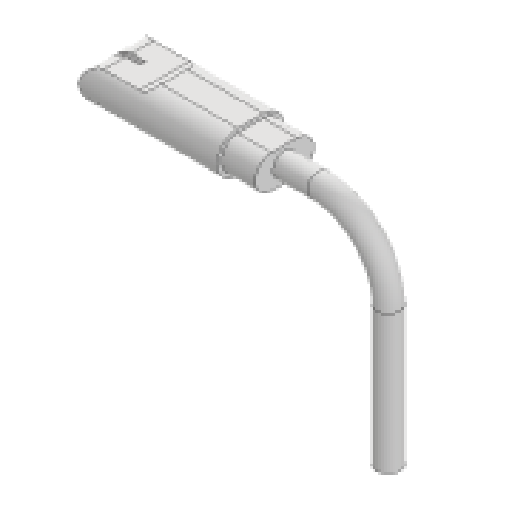
# Autodesk Inventor part: 基座
Saved by Autodesk Inventor 2025.2 (Build 292293000, 293)
## iProperties
Created: 2025-07-22
Part Number: 基座
Material: 一般
Document SubType Name: Modeling
Designer: jna1j
Density: 1 g/cm^3
Appearance: 預設
Author: jna1j
Autodesk Inventor part; units mm, degrees
ref_plane "YZ Plane" through (0, 0, 0) normal (1, 0, 0) x (0, 1, 0)
ref_plane "XZ Plane" through (0, 0, 0) normal (0, 1, 0) x (-1, 0, 0)
ref_plane "XY Plane" through (0, 0, 0) normal (0, 0, 1) x (1, 0, 0)
sketch "草圖1" plane through (0, 0, 0) normal (1, 0, 0) x (0, 1, 0)
  line L0 (-2.97, -1.859) -> (2.97, -1.859)
  line L1 (2.97, -1.859) -> (2.97, 1.859)
  line L2 (2.97, 1.859) -> (-2.97, 1.859)
  line L3 (-2.97, 1.859) -> (-2.97, -1.859)
  line L4 (-2.97, -1.859) -> (2.97, 1.859) construction
  line L5 (2.97, -1.859) -> (-2.97, 1.859) construction
  circle A0 centre (0, 1.859) radius 2.97
  circle A1 centre (0, -1.859) radius 2.97
  line L6 (-2.2651, -3.78) -> (-2.2651, 3.78) construction
  point P0 (0, 0)
  point P1 (-2.97, 1.859)
  dimension "d0" = 7.56
  dimension "d1" = 5.94
  constraints: 14 end point, 4 midpoint, 4 point on circle, 2 centre point, 2 parallel, 1 horizontal, 1 perpendicular, 1 vertical
  measures "d0" distance of L6.start L6.end
  measures "d1" distance of L1.end L2.end
extrude "擠出1" add sketch "草圖1" along normal blind 20
sketch "草圖2" plane through (0, 0, 0) normal (0, 0, 1) x (1, 0, 0)
  line L0 (0, 2.4) -> (9, 2.4)
  line L1 (9, 2.4) -> (9, -2.4)
  line L2 (9, -2.4) -> (0, -2.4)
  line L3 (0, -2.4) -> (0, 2.4)
  line L4 (0, -2.97) -> (0, 2.97) projected
  circle A0 centre (2.4, 0) radius 2.4
  line L5 (9, 5) -> (20, 5)
  line L6 (20, 5) -> (20, -5)
  line L7 (20, -5) -> (9, -5)
  line L8 (9, -5) -> (9, 5)
  line L9 (0, -2.97) -> (0, 2.97) projected
  line L10 (0, 2.97) -> (20, 2.97) projected
  line L11 (20, -2.97) -> (20, 2.97) projected
  line L12 (0, -2.97) -> (20, -2.97) projected
  arc A1 (7.6018, 2.4) -> (9, 2.97) centre (7.6018, 4.4) ccw
  arc A2 (9, -2.97) -> (7.6018, -2.4) centre (7.6018, -4.4) ccw
  point P0 (0, 0)
  point P1 (0, 0)
  point P2 (9, 0)
  point P3 (2.4, 2.4)
  point P4 (2.4, -2.4)
  dimension "d4" = 4.8
  dimension "d5" = 9
  dimension "d6" = 2
  dimension "d7" = 2
  constraints: 16 end point, 6 point on line, 5 tangent, 4 midpoint, 4 parallel, 4 point on circle, 3 centre point, 2 horizontal, 2 perpendicular
  measures "d4" distance of L2.end L0.start
  measures "d5" distance of L1.end L2.end
  measures "d6" radius of A2
  measures "d7" radius of A1
extrude "擠出2" cut sketch "草圖2" along normal mid plane 20 contours A1 L8 L0 | L0 L1 L2 A0 | L8 L10 L6 L12 L1 | A0 | L8 L5 L6 L10 | L8 A2 L2 | L12 L6 L7 L8 keep common part
sketch "草圖3" plane through (0, 0, 0) normal (0, 0, 1) x (1, 0, 0)
  line L0 (-0.1991, -1.7797) -> (-0.0573, 1.9709) projected
  arc A0 (-0.1991, -1.7797) -> (-0.0573, 1.9709) centre (2.4, 0) ccw projected
  point P0 (0, 0)
extrude "擠出3" cut sketch "草圖3" along normal mid plane 0.84
sketch "草圖4" plane through (20, 0, 0) normal (1, 0, 0) x (0, 0, -1)
  line L0 (1.859, 2.97) -> (-1.859, 2.97) projected
  arc A0 (-1.859, 2.97) -> (-1.859, -2.97) centre (-1.859, 0) ccw projected
  line L1 (-1.859, -2.97) -> (1.859, -2.97) projected
  arc A1 (1.859, -2.97) -> (1.859, 2.97) centre (1.859, 0) ccw projected
  line L2 (1.859, 2.38) -> (-1.859, 2.38)
  arc A2 (-1.859, 2.38) -> (-1.859, -2.38) centre (-1.859, 0) ccw
  line L3 (-1.859, -2.38) -> (1.859, -2.38)
  arc A3 (1.859, -2.38) -> (1.859, 2.38) centre (1.859, 0) ccw
  point P0 (0, 0)
  dimension "d14" = 0.59
  constraints: 4 end point, 4 point on circle, 2 centre point, 3 other
  measures "d14" radial gap between concentric circles of A1 A3
extrude "擠出4" add sketch "草圖4" along normal blind 4.88 contours A3 L3 A2 L2
sketch "草圖5" plane through (24.88, 0, 0) normal (1, 0, 0) x (0, 0, -1)
  circle A0 centre (0, 0) radius 1.7
  dimension "d17" = 3.4
  constraints: 1 centre point, 1 coincident
  measures "d17" diameter of A0
sketch "草圖6" plane through (0, 0, 0) normal (0, 0, 1) x (1, 0, 0)
  line L0 (24.88, -1.7) -> (24.88, 1.7) projected
  line L1 (24.88, 0) -> (29.88, 0)
  arc A0 (39.88, -10) -> (29.88, 0) centre (29.88, -10) ccw
  line L2 (39.88, -10) -> (39.88, -30)
  point P0 (0, 0)
  dimension "d18" = 5
  dimension "d19" = 10
  dimension "d20" = 20
  constraints: 4 end point, 2 point on circle, 2 tangent, 1 centre point, 1 horizontal, 1 midpoint, 1 vertical
  measures "d18" distance of L1.start L1.end
  measures "d19" radius of A0
  measures "d20" distance of L2.start L2.end
sweep "掃掠1" add profiles "草圖5" path "草圖6" path curves L1 A0 L2
